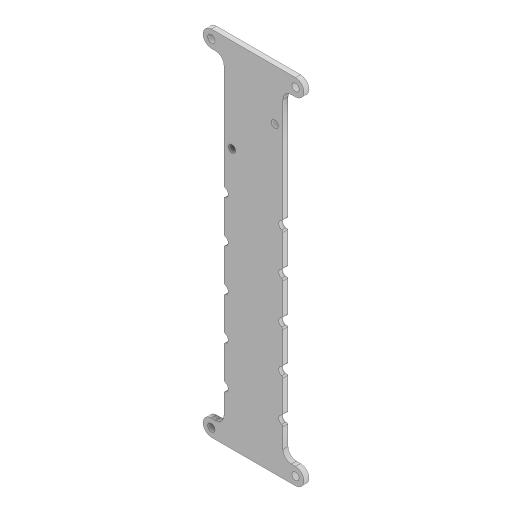
# Autodesk Inventor part: rx_frontend_generic
Saved by Autodesk Inventor 2023 (Build 270158000, 158)
## iProperties
Created: 2024-05-13
Part Number: rx_frontend_generic
Material: Generic
Document SubType Name: Modeling
Designer: Thomas
Density: 1 g/cm^3
Appearance: Default
Author: Thomas
Autodesk Inventor part; units mm, degrees
ref_plane "YZ Plane" through (0, 0, 0) normal (1, 0, 0) x (0, 1, 0)
ref_plane "XZ Plane" through (0, 0, 0) normal (0, 1, 0) x (-1, 0, 0)
ref_plane "XY Plane" through (0, 0, 0) normal (0, 0, 1) x (1, 0, 0)
sketch "Sketch1" plane through (0, 0, 0) normal (0, 0, 1) x (1, 0, 0)
  circle A0 centre (0, 0) radius 2.2
  line L0 (7.5, 0) -> (42.5, 0)
  line L1 (42.5, 0) -> (42.5, 200)
  line L2 (42.5, 200) -> (7.5, 200)
  line L3 (7.5, 200) -> (7.5, 0)
  circle A1 centre (50, 0) radius 2.2
  circle A2 centre (0, 200) radius 2.2
  circle A3 centre (50, 200) radius 2.2
  line L4 (0, 0) -> (50, 0) construction
  line L5 (0, -5) -> (50, -5)
  line L6 (50, 5) -> (0, 5)
  arc A4 (0, 5) -> (0, -5) centre (0, 0) ccw
  arc A5 (50, -5) -> (50, 5) centre (50, 0) ccw
  line L7 (0, 200) -> (50, 200) construction
  line L8 (0, 195) -> (50, 195)
  line L9 (50, 205) -> (0, 205)
  arc A6 (0, 205) -> (0, 195) centre (0, 200) ccw
  arc A7 (50, 195) -> (50, 205) centre (50, 200) ccw
  point P0 (25, 0)
  point P1 (25, 0)
  point P2 (25, 200)
  point P3 (7.5, 5)
  point P4 (42.5, 5)
  point P5 (42.5, 195)
  point P6 (7.5, 195)
  dimension "d0" = 4.4
  dimension "d1" = 35
  dimension "d2" = 200
  dimension "d3" = 25
  dimension "d5" = 0
  dimension "d8" = 50
  dimension "d11" = 200
  dimension "d14" = 10
  dimension "d15" = 10
  constraints: 24 end point, 8 centre point, 8 point on circle, 8 tangent, 5 parallel, 3 midpoint, 2 horizontal, 1 coincident, 1 collinear, 1 perpendicular, 1 vertical, 6 other
  measures "d0" diameter of A0
  measures "d1" distance of L2.end L1.end
  measures "d2" distance of L1.end L0.end
  measures "d3" distance of point (0, 0) point (25, 0)
  measures "d5" distance from line of L0 point (0, 0)
  measures "d8" distance of L4.start L4.end
  measures "d11" distance of L4.start L7.start
  measures "d14" diameter of A5
  measures "d15" diameter of A7
extrude "Extrusion1" add sketch "Sketch1" against normal blind 3
fillet "Fillet1" radius 5 4 edges at (7.5, 5, -1.5) (42.5, 5, -1.5) (42.5, 195, -1.5) (7.5, 195, -1.5)
sketch "Sketch2" plane through (0, 0, 0) normal (0, 0, 1) x (1, 0, 0)
  circle A0 centre (0, 200) radius 2.2 projected
  circle A1 centre (50, 200) radius 2.2 projected
  line L0 (0, 200) -> (50, 200) construction
  circle A2 centre (37.7, 175) radius 2.1
  circle A3 centre (12.3, 149.6) radius 2.1
  line L1 (37.7, 175) -> (12.3, 175) construction
  line L2 (12.3, 175) -> (12.3, 149.6) construction
  line L3 (12.3, 149.6) -> (37.7, 149.6) construction
  line L4 (37.7, 149.6) -> (37.7, 175) construction
  point P0 (0, 0)
  point P1 (25, 200)
  point P2 (25, 175)
  dimension "d19" = 4.2
  dimension "d20" = 4.2
  dimension "d21" = 25
  dimension "d22" = 25.4
  dimension "d23" = 25.4
  dimension "d24" = 0
  constraints: 10 end point, 2 centre point, 2 horizontal, 2 midpoint, 2 parallel, 1 perpendicular
  measures "d19" diameter of A2
  measures "d20" diameter of A3
  measures "d21" distance from line of L1.start L0
  measures "d22" distance of L1.start L1.end
  measures "d23" distance of L1.end L2.end
  measures "d24" horizontal distance of point (25, 200) point (25, 175)
extrude "Extrusion2" cut sketch "Sketch2" against normal blind 3 contours A2 | A3
sketch "Sketch3" plane through (0, 0, 0) normal (0, 0, 1) x (1, 0, 0)
  line L0 (7.5, 10) -> (7.5, 190) projected
  circle A0 centre (7.5, 25) radius 2.5
  line L1 (42.5, 190) -> (42.5, 10) projected
  circle A1 centre (42.5, 25) radius 2.5
  point P0 (0, 0)
  point P1 (42.5, 22.5)
  point P2 (42.5, 27.5)
  point P3 (7.5, 27.5)
  point P4 (7.5, 22.5)
  dimension "d27" = 5
  dimension "d28" = 25
  dimension "d29" = 5
  dimension "d30" = 25
  constraints: 2 centre point, 2 point on line
  measures "d27" diameter of A0
  measures "d28" vertical distance of point (0, 0) A0.centre
  measures "d29" diameter of A1
  measures "d30" vertical distance of point (0, 0) A1.centre
extrude "Extrusion3" cut sketch "Sketch3" against normal blind 3 contours L0 A0 | L1 A1 picked at (8.4362, 25.3407) picked at (41.0396, 24.5266)
fillet "Fillet2" radius 1 6 edges at (7.5, 22.5, -1.5) (7.5, 27.5, -1.5) (42.5, 27.5, -1.5) (42.5, 22.5, -1.5) (40, 25, -3) (10, 25, -3)
pattern_linear "Rectangular Pattern1" count 5 spacing 25 along (0, 1, 0) of "Extrusion3", "Fillet2"
equation "\"d20\" = d19"
body "Solid1"
